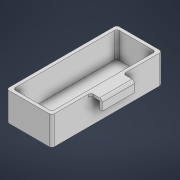
# Autodesk Inventor part: AccesoryHolder
Saved by Autodesk Inventor 2022 (Build 260153000, 153)
## iProperties
Created: 2024-01-20
Part Number: AccesoryHolder
Material: Všeobecné
Document SubType Name: Modeling
Designer: tada
Density: 1 g/cm^3
Appearance: Výchozí
Author: tada
Autodesk Inventor part; units mm, degrees
ref_plane "YZ Plane" through (0, 0, 0) normal (1, 0, 0) x (0, 1, 0)
ref_plane "XZ Plane" through (0, 0, 0) normal (0, 1, 0) x (-1, 0, 0)
ref_plane "XY Plane" through (0, 0, 0) normal (0, 0, 1) x (1, 0, 0)
sketch "Náčrt1" plane through (0, 0, 0) normal (0, 1, 0) x (-1, 0, 0)
  line L0 (0, 0) -> (-30, 0)
  line L1 (-30, 0) -> (-30, -80)
  line L2 (-30, -80) -> (0, -80)
  line L3 (0, -80) -> (0, 0)
  line L4 (2.5, 2.5) -> (-32.5, 2.5)
  line L5 (-32.5, 2.5) -> (-32.5, -82.5)
  line L6 (-32.5, -82.5) -> (2.5, -82.5)
  line L7 (2.5, -82.5) -> (2.5, 2.5)
  dimension "d0" = 80
  dimension "d1" = 30
  dimension "d2" = 2.5
  constraints: 16 end point, 4 parallel, 2 perpendicular, 1 horizontal, 3 other
  measures "d0" distance of L2.end L0.start
  measures "d1" distance of L1.end L2.end
  measures "d2" distance between parallel lines of L7 L3
extrude "Vysunutí1" add sketch "Náčrt1" along normal blind 2 contours L3 L2 L1 L0
extrude "Vysunutí2" add sketch "Náčrt1" along normal blind 22
sketch "Náčrt2" plane through (32.5, 0, 2.5) normal (1, 0, 0) x (0, 0, -1)
  line L0 (0, 22) -> (85, 22) projected
  line L1 (30, 22) -> (55, 22)
  line L2 (55, 22) -> (55, 20)
  line L3 (55, 20) -> (30, 20)
  line L4 (30, 20) -> (30, 22)
  line L5 (85, 0) -> (85, 22) projected
  line L6 (0, 0) -> (0, 22) projected
  point P0 (2.5, 0)
  dimension "d7" = 30
  dimension "d8" = 30
  dimension "d9" = 2
  constraints: 8 end point, 2 parallel, 1 horizontal, 1 perpendicular, 1 point on line
  measures "d7" distance between parallel lines of L5 L2
  measures "d8" distance between parallel lines of L6 L4
  measures "d9" distance between parallel lines of L3 L0
extrude "Vysunutí3" add sketch "Náčrt2" along normal blind 8.8
sketch "Náčrt3" plane through (32.5, 20, -52.5) normal (0, -1, 0) x (1, 0, 0)
  line L0 (0, 25) -> (8.8, 25) projected
  line L1 (0, 0) -> (8.8, 0) projected
  line L2 (8.8, 25) -> (6.8, 25)
  line L3 (6.8, 25) -> (6.8, 0)
  line L4 (6.8, 0) -> (8.8, 0)
  line L5 (8.8, 0) -> (8.8, 25)
  point P0 (-32.5, 52.5)
  point P1 (8.8, 0)
  point P2 (6.8, 25)
  dimension "d12" = 2
  constraints: 8 end point, 2 parallel, 1 horizontal, 1 perpendicular, 1 point on line
  measures "d12" distance between parallel lines of L5 L3
extrude "Vysunutí4" add sketch "Náčrt3" along normal blind 6
fillet "Zaoblení1" radius 2 3 edges at (41.3, 22, -40) (32.5, 21, -52.5) (32.5, 21, -27.5)
fillet "Zaoblení2" radius 2 4 edges at (-2.5, 11, 2.5) (32.5, 11, 2.5) (32.5, 11, -82.5) (-2.5, 11, -82.5)
fillet "Zaoblení3" radius 2 4 edges at (30, 12, -80) (30, 12, 0) (0, 12, -80) (0, 12, 0)
equation "\"d8\" = d7"
